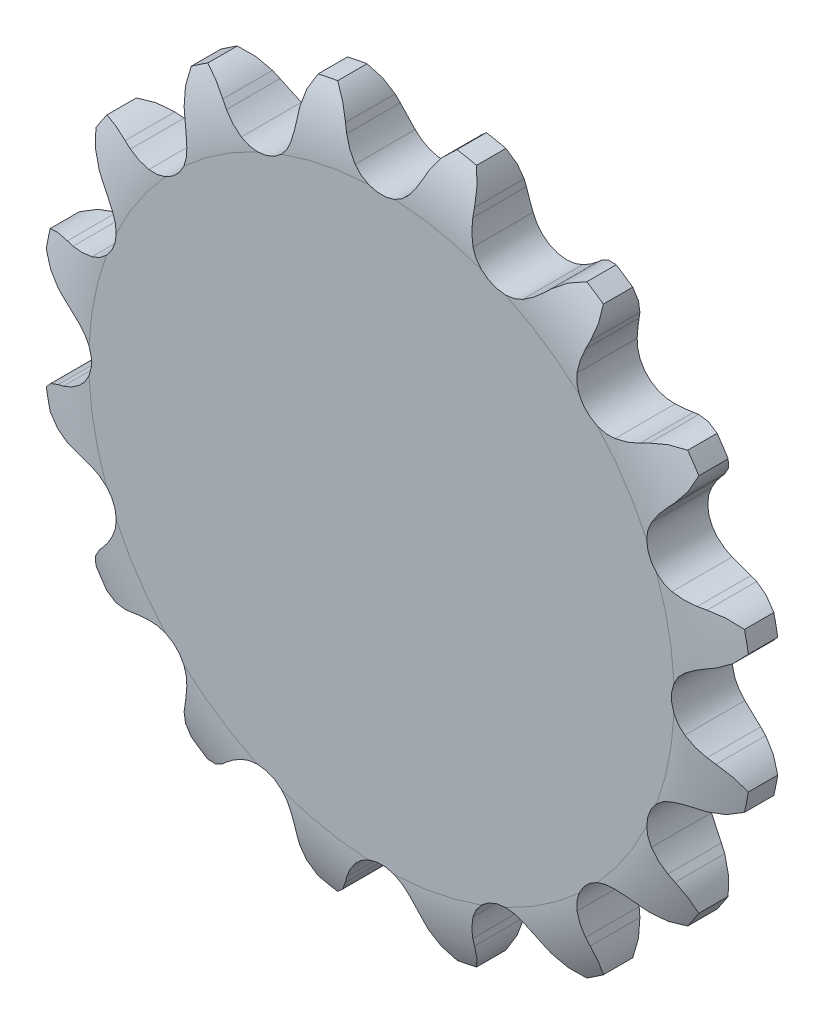
# Autodesk Inventor part: Roller Chain Sprocket2
Saved by Autodesk Inventor 2016 SP1 (Build 200210100, 210)
## iProperties
Created: 2016-02-02
Part Number: Roller Chain Sprocket2
Material: Steel
Document SubType Name: Modeling
Designer: steele
Density: 7.85 g/cm^3
Appearance: Steel
Mass: 64.065 g
Surface Area: 45.5226 cm^2
Volume: 8.16115 cm^3
CustomPartVersion: 1
Author: steele
Autodesk Inventor part; units mm, degrees
ref_plane "YZ Plane" through (0, 0, 0) normal (1, 0, 0) x (0, 1, 0)
ref_plane "XZ Plane" through (0, 0, 0) normal (0, 1, 0) x (-1, 0, 0)
ref_plane "XY Plane" through (0, 0, 0) normal (0, 0, 1) x (1, 0, 0)
sketch "Theoretical Tooth Profile" plane through (0, 0, 0) normal (0, 0, 1) x (1, 0, 0)
  circle A0 centre (0, 0) radius 24.4118 construction
  line L0 (0, 0) -> (0, 24.4118) construction
  line L1 (0, 0) -> (9.342, 22.5535) construction
  circle A1 centre (0, 0) radius 26.8002
  arc A2 (-2.0205, 22.7901) -> (2.0205, 22.7901) centre (0, 24.4118) ccw
  line L2 (0, 24.4118) -> (9.342, 22.5535) construction
  line L3 (0, 24.4118) -> (3.1695, 26.9555) construction
  line L4 (3.1695, 26.9555) -> (-2.8981, 24.2223) construction
  arc A3 (4.4896, 26.4215) -> (3.1373, 24.7532) centre (6.9753, 23.0243) ccw
  arc A4 (-3.1373, 24.7532) -> (-4.4896, 26.4215) centre (-6.9753, 23.0243) ccw
  line L5 (-6.9753, 23.0243) -> (-3.1373, 24.7532) construction
  arc A5 (-2.8981, 24.2223) -> (-2.0205, 22.7901) centre (3.1695, 26.9555) ccw
  line L6 (-2.8981, 24.2223) -> (-3.1373, 24.7532)
  arc A6 (2.0205, 22.7901) -> (2.8981, 24.2223) centre (-3.1695, 26.9555) ccw
  line L7 (3.1373, 24.7532) -> (2.8981, 24.2223)
  line L8 (0, 0) -> (5.2285, 26.2852) construction
  point P0 (4.671, 23.4827)
  dimension "d0" = 48.8235
  dimension "d2" = 22.5
  dimension "d3" = 2.5908
  dimension "d10" = 128.75
  dimension "d11" = 14.5
  dimension "d12" = 4.064
  dimension "d13" = 6.6548
  dimension "d14" = 7.112
  dimension "d23" = 2.8575
  constraints: 18 end point, 15 point on circle, 7 centre point, 3 coincident, 3 point on line, 3 symmetric about line, 3 tangent, 1 equal radius, 1 midpoint, 1 parallel, 1 vertical, 1 other
  measures "d0" diameter of A0
  measures "d2" angle of L1 L0
  measures "d3" radius of A2
  measures "d10" angle of L3 L0
  measures "d11" angle of L4 L3
  measures "d12" distance of L2.start L3.end
  measures "d13" distance of L3.end L4.end
  measures "d14" distance of A3.centre L0.end
  measures "d23" distance from line of L8.end L2
sketch "Tooth Profile" plane through (0, 0, 0) normal (0, 0, 1) x (1, 0, 0)
  circle A0 centre (0, 0) radius 26.8002 projected
  line L0 (0, 0) -> (0, 24.4118) construction
  line L1 (0, 24.4118) -> (2.3881, 23.4073) construction
  arc A1 (-2.3881, 23.4073) -> (2.3881, 23.4073) centre (0, 24.4118) ccw
  line L2 (-2.3881, 23.4073) -> (0, 24.4118) construction
  arc A2 (-2.3881, 23.4073) -> (-4.3092, 26.4515) centre (-12.5026, 19.1529) ccw
  arc A3 (4.3092, 26.4515) -> (2.3881, 23.4073) centre (12.5026, 19.1529) ccw
  dimension "d44" = 134.375
  dimension "d45" = 2.5908
  dimension "d46" = 10.9728
  constraints: 8 point on circle, 7 end point, 3 centre point, 2 tangent, 1 coincident, 1 equal radius, 1 symmetric about line, 1 vertical
  measures "d44" angle of L1 L2
  measures "d45" radius of A1
  measures "d46" radius of A3
sketch "Section Profile" plane through (0, 0, 0) normal (1, 0, 0) x (0, 1, 0)
  line L0 (26.8002, 0) -> (-26.8002, 0) projected
  line L1 (18.4182, 2.2967) -> (-18.4182, 2.2967)
  line L2 (-18.4182, 2.2967) -> (-18.4182, -2.2967)
  line L3 (-18.4182, -2.2967) -> (18.4182, -2.2967)
  line L4 (18.4182, -2.2967) -> (18.4182, 2.2967)
  line L5 (18.4182, 2.2967) -> (26.8002, 2.2967) construction
  line L6 (26.8002, 2.2967) -> (26.8002, -2.2967) construction
  line L7 (26.8002, -2.2967) -> (18.4182, -2.2967) construction
  line L8 (18.4182, -2.2967) -> (18.4182, 2.2967)
  arc A0 (26.8002, 1.106) -> (22.0365, 2.2967) centre (22.0365, -7.8284) ccw
  arc A1 (22.0365, -2.2967) -> (26.8002, -1.106) centre (22.0365, 7.8284) ccw
  line L9 (22.0365, 2.2967) -> (0, 2.2967)
  line L10 (0, 2.2967) -> (0, -2.2967)
  line L11 (0, -2.2967) -> (22.0365, -2.2967)
  line L12 (0, 2.2967) -> (0, -2.2967)
  line L13 (26.8002, 1.106) -> (26.8002, -1.106)
  point P0 (0, 0)
  point P1 (0, 0)
  dimension "d30" = 4.5933
  dimension "d31" = 36.8364
  dimension "d32" = 4.5933
  dimension "d33" = 1.1906
  dimension "d34" = 10.1251
  dimension "d43" = 2.2967
  constraints: 26 end point, 7 midpoint, 5 perpendicular, 4 parallel, 4 point on circle, 3 point on line, 3 symmetric about line, 2 centre point, 2 horizontal, 2 tangent, 1 collinear, 1 other
  measures "d30" distance between parallel lines of L7 L5
  measures "d31" distance between parallel lines of L2 L4
  measures "d32" distance between parallel lines of L3 L1
  measures "d33" distance from line of L13.start L5
  measures "d34" radius of A0
  measures "d43" distance between parallel lines of L3 L0
revolve "Shroud" add sketch "Section Profile" angle 360 about axis through (0, 0, 2.2967) along (0, 0, -1) contours L10 L3 L2 L0 | L0 L2 L1 L10
revolve "Strand" add sketch "Section Profile" angle 360 about axis through (0, 0, 2.2967) along (0, 0, -1) contours L13 A1 L11 L4 L0 | L0 L4 L9 A0 L13 | L4 L3 L10 L0 | L0 L10 L1 L4
pattern_of_one "Strand Pattern"
extrude "Theoretical Tooth" cut sketch "Theoretical Tooth Profile" along normal through all both and the other way through all contours A3 L7 A6 A2 A5 L6 A4 A1 picked at (0.5009, 24.1127)
extrude "Tooth" [suppressed]
pattern_circular "Tooth Pattern" count 16 over 360 about axis through (0, 0, -10) along (0, 0, 1) of "Theoretical Tooth"
ref_plane "Timing Plane" through (0, 24.4118, 0) normal (1, 0, 0) x (0, 1, 0)
equation "\"d3\" = 0.5 * da_Dr + da_SC"
equation "\"d12\" = 0.8 * da_Dr"
equation "\"d13\" = 1.3 * da_Dr + da_SC"
equation "\"d14\" = 1.4 * da_Dr"
equation "\"d23\" = da_Ha"
equation "\"d44\" = da_Alfa"
equation "\"d45\" = da_Ri"
equation "\"d46\" = da_Re"
equation "\"d30\" = da_Bf"
equation "\"d31\" = da_Ds"
equation "\"d32\" = da_Bs"
equation "\"d33\" = da_Ba"
equation "\"d34\" = da_Rx"
equation "\"d40\" = da_pt"
equation "\"form_type\" = 0"
equation "\"da_p\" = 9.525"
equation "\"da_Dr\" = 5.08"
equation "\"da_SC\" = 0.0508"
equation "\"da_Ha\" = 2.8575"
equation "\"da_pt\" = 10.1346"
equation "\"da_Bf\" = 4.59334"
equation "\"da_Ba\" = 1.19063"
equation "\"da_Rx\" = 10.12508"
equation "\"da_Ra\" = 0.381"
equation "\"da_Bs\" = 4.59334"
equation "\"da_Ds\" = 36.83641"
equation "\"da_Re\" = 10.9728"
equation "\"da_Ri\" = 2.5908"
equation "\"da_Alfa\" = 134.375deg"
body "Solid1"
